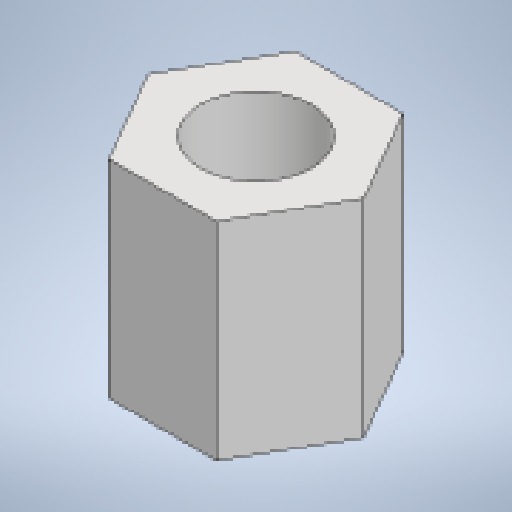
# Autodesk Inventor part: hexstandoff
Saved by Autodesk Inventor 2026 (Build 300175050, 175E)
## iProperties
Created: 2025-12-28
Part Number: hexstandoff
Material: Nylon 6/6
Document SubType Name: Modeling
Designer: Nicholas M
Density: 1.13 g/cm^3
Appearance: Smooth - Black
Author: Nicholas M
Autodesk Inventor part; units mm, degrees
ref_plane "YZ Plane" through (0, 0, 0) normal (1, 0, 0) x (0, 1, 0)
ref_plane "XZ Plane" through (0, 0, 0) normal (0, 1, 0) x (-1, 0, 0)
ref_plane "XY Plane" through (0, 0, 0) normal (0, 0, 1) x (1, 0, 0)
sketch "Sketch1" plane through (0, 0, 0) normal (0, 1, 0) x (-1, 0, 0)
  line L0 (1.5588, -2.7) -> (-1.5588, -2.7)
  line L1 (-1.5588, -2.7) -> (-3.1177, 0)
  line L2 (-3.1177, 0) -> (-1.5588, 2.7)
  line L3 (-1.5588, 2.7) -> (1.5588, 2.7)
  line L4 (1.5588, 2.7) -> (3.1177, 0)
  line L5 (3.1177, 0) -> (1.5588, -2.7)
  circle A0 centre (0, 0) radius 1.6
  dimension "d0" = 5.4
  dimension "d1" = 3.2
  constraints: 12 end point, 2 coincident, 1 centre point, 1 horizontal, 13 other
  measures "d0" distance between parallel lines of L2 L5
  measures "d1" diameter of A0
extrude "Extrusion1" add sketch "Sketch1" along normal blind 6
body "Solid1"
